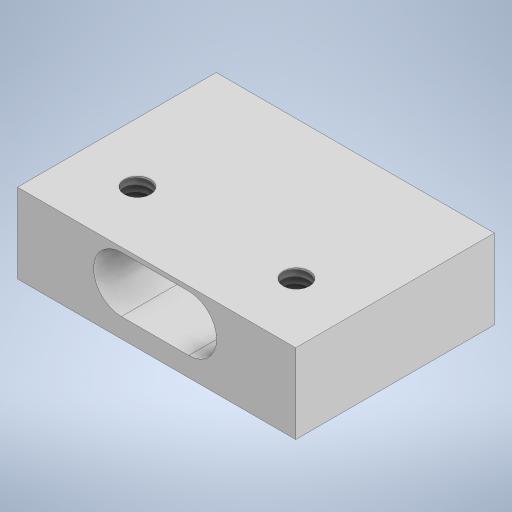
# Autodesk Inventor part: ResonantAdapter
Saved by Autodesk Inventor 2023 (Build 270158000, 158)
## iProperties
Created: 2024-01-12
Part Number: ResonantAdapter
Material: Generic
Document SubType Name: Modeling
Designer: kerlin
Density: 1 g/cm^3
Appearance: Default
Author: kerlin
Autodesk Inventor part; units mm, degrees
ref_plane "YZ Plane" through (0, 0, 0) normal (1, 0, 0) x (0, 1, 0)
ref_plane "XZ Plane" through (0, 0, 0) normal (0, 1, 0) x (-1, 0, 0)
ref_plane "XY Plane" through (0, 0, 0) normal (0, 0, 1) x (1, 0, 0)
sketch "Sketch1" plane through (0, 0, 0) normal (0, 1, 0) x (-1, 0, 0)
  line L0 (12.5, 12.5) -> (-12.5, 12.5)
  line L1 (-12.5, 12.5) -> (-12.5, -12.5)
  line L2 (-12.5, -12.5) -> (12.5, -12.5)
  line L3 (12.5, -12.5) -> (12.5, 12.5)
  line L4 (12.5, 12.5) -> (-12.5, -12.5) construction
  line L5 (-12.5, 12.5) -> (12.5, -12.5) construction
  point P0 (0, 0)
  dimension "d0" = 25
  dimension "d1" = 25
  constraints: 12 end point, 2 midpoint, 2 parallel, 1 horizontal, 1 perpendicular
  measures "d0" distance of L2.end L0.start
  measures "d1" distance of L1.end L2.end
extrude "Extrusion1" add sketch "Sketch1" along normal blind 10
sketch "Sketch2" plane through (-12.5, 0, 12.5) normal (0, 0, 1) x (1, 0, 0)
  line L0 (25, 0) -> (25, 10) projected
  line L1 (0, 10) -> (25, 10) projected
  point P0 (12.5, 0)
  point P1 (12.5, 5.936)
  dimension "d12" = 4.064
  measures "d12" distance from line of L1 point (12.5, 5.936)
hole "Hole1" at (0, 5.936, 12.5) direction (0, 0, -1) diameter 5 depth 25 counterbore diameter 7 counterbore depth 20
sketch "Sketch4" plane through (-12.5, 0, 12.5) normal (0, 0, 1) x (1, 0, 0)
  line L0 (4.5617, 5.936) -> (20.0475, 5.936) construction
  line L1 (8.0617, 9.436) -> (16.5475, 9.436)
  line L2 (16.5475, 2.436) -> (8.0617, 2.436)
  arc A0 (8.0617, 9.436) -> (8.0617, 2.436) centre (8.0617, 5.936) ccw
  arc A1 (16.5475, 2.436) -> (16.5475, 9.436) centre (16.5475, 5.936) ccw
  point P0 (12.5, 0)
  point P1 (12.3046, 5.936)
  constraints: 8 end point, 6 point on circle, 4 tangent, 2 centre point, 2 point on line, 1 horizontal, 1 midpoint, 1 parallel
extrude "Extrusion2" cut sketch "Sketch4" against normal blind 20
sketch "Sketch5" plane through (-4.4383, 9.436, -7.5) normal (0, 0, 1) x (1, 0, 0)
  line L0 (-2.0833, -3.5) -> (10.4225, -3.5) construction
  line L1 (0.4167, -1) -> (7.9225, -1)
  line L2 (7.9225, -6) -> (0.4167, -6)
  arc A0 (0.4167, -1) -> (0.4167, -6) centre (0.4167, -3.5) ccw
  arc A1 (7.9225, -6) -> (7.9225, -1) centre (7.9225, -3.5) ccw
  point P0 (4.4383, -9.436)
  point P1 (4.1696, -3.5)
  constraints: 8 end point, 6 point on circle, 4 tangent, 2 centre point, 2 point on line, 1 horizontal, 1 midpoint, 1 parallel
extrude "Extrusion3" cut sketch "Sketch5" against normal blind 20
sketch "Sketch6" plane through (-12.5, 0, -12.5) normal (-1, 0, 0) x (0, 0, 1)
  line L0 (25, 10) -> (0, 10) projected
  line L1 (0, 0) -> (25, 0) projected
  line L2 (0, 10) -> (25, 10)
  line L3 (25, 10) -> (25, 0)
  line L4 (25, 0) -> (0, 0)
  line L5 (0, 0) -> (0, 10)
  point P0 (12.5, 0)
  constraints: 8 end point, 2 parallel, 1 horizontal, 1 perpendicular
extrude "Extrusion4" add sketch "Sketch6" along normal blind 5
sketch "Sketch7" plane through (12.5, 0, 12.5) normal (1, 0, 0) x (0, 0, -1)
  line L0 (0, 10) -> (25, 10) projected
  line L1 (0, 0) -> (25, 0) projected
  line L2 (0, 10) -> (25, 10)
  line L3 (25, 10) -> (25, 0)
  line L4 (25, 0) -> (0, 0)
  line L5 (0, 0) -> (0, 10)
  point P0 (12.5, 0)
  constraints: 8 end point, 2 parallel, 1 horizontal, 1 perpendicular
extrude "Extrusion5" add sketch "Sketch7" along normal blind 5
sketch "Sketch8" plane through (0, 10, 0) normal (0, 1, 0) x (1, 0, 0)
  line L0 (-17.5, 12.5) -> (17.5, 12.5) projected
  line L1 (-17.5, -12.5) -> (-17.5, 12.5) projected
  line L2 (17.5, 12.5) -> (17.5, -12.5) projected
  point P0 (0, 0)
  point P1 (10, -4.917)
  point P2 (-10, -4.917)
  dimension "d28" = 17.417
  dimension "d29" = 17.417
  dimension "d30" = 7.5
  dimension "d31" = 7.5
  measures "d28" distance from line of L0 point (-10, -4.917)
  measures "d29" distance from line of L0 point (10, -4.917)
  measures "d30" distance from line of point (-10, -4.917) L1
  measures "d31" distance from line of L2 point (10, -4.917)
hole "Hole2" at (10, 10, 4.917) at (-10, 10, 4.917) direction (0, -1, 0) diameter 3.302 depth 12.3 thread size "8-32 UNC" class "2B" standard "ANSI Unified Screw Threads"
body "Solid1"
